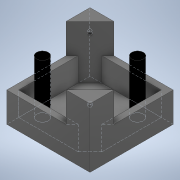
# Autodesk Inventor part: disk holder
Saved by Autodesk Inventor 2022 (Build 260153000, 153)
## iProperties
Created: 2022-02-07
Part Number: disk holder
Material: ABS Plastic
Document SubType Name: Modeling
Designer: joshw
Density: 1.06 g/cm^3
Appearance: Smooth - White
Author: joshw
Autodesk Inventor part; units mm, degrees
ref_plane "YZ Plane" through (0, 0, 0) normal (1, 0, 0) x (0, 1, 0)
ref_plane "XZ Plane" through (0, 0, 0) normal (0, 1, 0) x (-1, 0, 0)
ref_plane "XY Plane" through (0, 0, 0) normal (0, 0, 1) x (1, 0, 0)
sketch "Sketch1" plane through (0, 0, 0) normal (0, 1, 0) x (-1, 0, 0)
  line L0 (7, 7) -> (-7, 7)
  line L1 (-7, 7) -> (-7, -7)
  line L2 (-7, -7) -> (7, -7)
  line L3 (7, -7) -> (7, 7)
  line L4 (7, 7) -> (-7, -7) construction
  line L5 (-7, 7) -> (7, -7) construction
  line L6 (6, 6) -> (-6, 6)
  line L7 (-6, 6) -> (-6, -6)
  line L8 (-6, -6) -> (6, -6)
  line L9 (6, -6) -> (6, 6)
  point P0 (0, 0)
  dimension "d0" = 14
  dimension "d1" = 14
  dimension "d2" = 1
  constraints: 20 end point, 4 parallel, 2 midpoint, 2 perpendicular, 1 horizontal, 3 other
  measures "d0" distance of L2.end L1.end
  measures "d1" distance of L1.end L0.end
  measures "d2" distance between parallel lines of L3 L9
extrude "Extrusion1" add sketch "Sketch1" along normal blind 5
sketch "Sketch2" plane through (0, 5, 0) normal (0, 1, 0) x (1, 0, 0)
  line L0 (-7, -7) -> (7, -7) projected
  line L1 (3, -7) -> (7, -3)
  line L2 (7, -7) -> (7, 7) projected
  line L3 (-7, 7) -> (-7, -7) projected
  line L4 (-7, 3) -> (-3, 7)
  line L5 (7, 7) -> (-7, 7) projected
  point P0 (0, 0)
  dimension "d5" = 4
  dimension "d6" = 4
  dimension "d7" = 4
  dimension "d8" = 4
  constraints: 4 end point, 4 point on line
  measures "d5" distance of L1.start L0.end
  measures "d6" distance of L1.end L0.end
  measures "d7" distance of L4.start L3.start
  measures "d8" distance of L4.end L3.start
extrude "Extrusion2" add sketch "Sketch2" along normal mid plane 10 contours L1 L2 L0 | L3 L5 L4
sketch "Sketch3" plane through (0, 0, 0) normal (0, -1, 0) x (1, 0, 0)
  line L0 (7, -7) -> (-7, -7) projected
  line L1 (7, 7) -> (7, -7) projected
  line L2 (-7, 7) -> (7, 7) projected
  line L3 (-7, -7) -> (-7, 7) projected
  line L4 (-4, -6) -> (-6, -4) projected
  line L5 (-6, 6) -> (-6, -4) projected
  line L6 (4, 6) -> (-6, 6) projected
  line L7 (4, 6) -> (6, 4) projected
  line L8 (6, -6) -> (6, 4) projected
  line L9 (-4, -6) -> (6, -6) projected
  point P0 (0, 0)
extrude "Extrusion3" add sketch "Sketch3" against normal blind 1 contours L0 L3 L2 L1 | L4 L5 L6 L7 L8 L9
sketch "Sketch4" plane through (0, 1, 0) normal (0, 1, 0) x (1, 0, 0)
  circle A0 centre (-4, -4) radius 0.9814
  circle A1 centre (4, 4) radius 0.9814
  line L0 (-6, -6) -> (-6, 4) projected
  line L1 (4, -6) -> (-6, -6) projected
  line L2 (-4, 6) -> (6, 6) projected
  line L3 (6, 6) -> (6, -4) projected
  point P0 (0, 0)
  dimension "d15" = 2
  dimension "d16" = 2
  dimension "d17" = 2
  dimension "d18" = 2
  constraints: 2 centre point, 1 equal radius
  measures "d15" distance from line of L0 A0.centre
  measures "d16" distance from line of L1 A0.centre
  measures "d17" distance from line of L2 A1.centre
  measures "d18" distance from line of L3 A1.centre
extrude "Extrusion4" add sketch "Sketch4" along normal blind 9
sketch "Sketch5" plane through (-3, 5, -7) normal (0.7071, 0, 0.7071) x (0.7071, 0, -0.7071)
  line L0 (-2.8284, -5) -> (-2.8284, 5) projected
  circle A0 centre (-2.8284, 3.1472) radius 0.25
  dimension "d19" = 0.5
  constraints: 1 centre point, 1 point on line
  measures "d19" diameter of A0
extrude "Extrusion5" cut sketch "Sketch5" along normal blind 14.75 and the other way blind 0.75
body "Solid1"
